# Autodesk Inventor part: 主动轮锥齿轮
Saved by Autodesk Inventor 2015 (Build 190159000, 159)
## iProperties
Created: 2017-06-08
Part Number: 主动轮锥齿轮
Material: 铝 6061
Document SubType Name: Modeling
Designer: Administrator
Categories: <?xml version="1.0" encoding="UTF-16"?> <MemberInstance><Categories><FamilyTemplate><FamilyTemplateParameter ValueType="xs:double" Id="1" ObjectReferenceKey="da_z" ObjectType="kUserParameterObject"/><FamilyTemplateParameter ValueType="xs:double" Id="2" ObjectReferenceKey="da_b" ObjectType="kUserParameterObject"/><FamilyTemplateParameter ValueType="xs:double" Id="3" ObjectReferenceKey="da_beta" ObjectType="kUserParameterObject"/><FamilyTemplateParameter ValueType="xs:double" Id="4" ObjectReferenceKey="da_dae" ObjectType="kUserParameterObject"/><FamilyTemplateParameter ValueType="xs:double" Id="5" ObjectReferenceKey="da_ve" ObjectType="kUserParameterObject"/><FamilyTemplateParameter ValueType="xs:double" Id="6" ObjectReferenceKey="da_omega" ObjectType="kUserParameterObject"/><FamilyTemplateParameter ValueType="xs:string" Id="7" ObjectReferenceKey="EAIAABAAAAAAHwAAAAAAAIAAAAAAAAAA" ObjectType="83914240" SubObjectId="SurfaceGeometry"/></FamilyTemplate><ParamToTemplateMap><ParamToTemplate CategoryParameter="//CategoryParameter[@InternalName='046C89C9-8512-4d59-83FE-43B91F4F132A']" TemplateParameter="1"/><ParamToTemplate CategoryParameter="//CategoryParameter[@InternalName='2552DF32-E462-4b46-AEBF-C6C7768E72AC']" TemplateParameter="2"/><ParamToTemplate CategoryParameter="//CategoryParameter[@InternalName='C9EE641D-15FC-4fae-A226-E94C4372FDD7']" TemplateParameter="3"/><ParamToTemplate><ParamToTemplate CategoryParameter="//CategoryParameter[@InternalName='00B6519A-459B-49c7-AD84-2E56D39A5744']" ConstantValue="0.000000"/></ParamToTemplate><ParamToTemplate><ParamToTemplate CategoryParameter="//CategoryParameter[@InternalName='04B31F0E-C7A6-4894-AA32-9629BEFACF47']" ConstantValue="1.000000"/></ParamToTemplate><ParamToTemplate><ParamToTemplate CategoryParameter="//CategoryParameter[@InternalName='43CBEC2E-7847-49e7-A936-2F7889FCB2D9']" ConstantValue="0.200000"/></ParamToTemplate><ParamToTemplate><ParamToTemplate CategoryParameter="//CategoryParameter[@InternalName='B1EFC894-105D-4ebd-86BF-FA20ED196853']" ConstantValue="0.300000"/></ParamToTemplate><ParamToTemplate><ParamToTemplate CategoryParameter="//CategoryParameter[@InternalName='51175063-3D10-4879-93E8-6246FE8B403D']" ConstantValue="2060000000.000000"/></ParamToTemplate><ParamToTemplate><ParamToTemplate CategoryParameter="//CategoryParameter[@InternalName='A3A52E27-4454-46a9-B0BD-C932399B70AF']" ConstantValue="0.300000"/></ParamToTemplate><ParamToTemplate CategoryParameter="//CategoryParameter[@InternalName='2A200944-5A8C-41ca-B96E-8520D2E510F1']" TemplateParameter="4"/><ParamToTemplate><ParamToTemplate CategoryParameter="//CategoryParameter[@InternalName='1A637F62-92C8-44bc-B81F-10802510B579']" ConstantValue="10.922917"/></ParamToTemplate><ParamToTemplate CategoryParameter="//CategoryParameter[@InternalName='B52DD4BE-6863-48fb-BF58-89EF6F9EC65C']" TemplateParameter="5"/><ParamToTemplate><ParamToTemplate CategoryParameter="//CategoryParameter[@InternalName='3956BFF2-84D2-457d-93C2-9B0613DEBA67']" ConstantValue="1.630592"/></ParamToTemplate><ParamToTemplate CategoryParameter="//CategoryParameter[@InternalName='739CFA02-461B-4bf8-8049-181FCAD8B28F']" TemplateParameter="6"/><ParamToTemplate><ParamToTemplate CategoryParameter="//CategoryParameter[@InternalName='A27E999F-E2CE-4481-8A2A-EBF499C4C3C5']" ConstantValue="0.000000"/></ParamToTemplate><ParamToTemplate><ParamToTemplate CategoryParameter="//CategoryParameter[@InternalName='9E1B4470-B2D3-4ff1-B813-535BB4CDF51A']" ConstantValue="3520000.000000"/></ParamToTemplate><ParamToTemplate><ParamToTemplate CategoryParameter="//CategoryParameter[@InternalName='F8452263-BFF6-458c-9FB1-07C4B99E95CD']" ConstantValue="11400000.000000"/></ParamToTemplate><ParamToTemplate><ParamToTemplate CategoryParameter="//CategoryParameter[@InternalName='3E3BB259-FD49-497f-8171-6EBC954A3479']" ConstantValue="2.000000"/></ParamToTemplate><ParamToTemplate CategoryParameter="//CategoryParameter[@InternalName='27C3BAF2-7550-4e4b-AE2C-0DB134B7D9B7']" TemplateParameter="7"/></ParamToTemplateMap><Category DisplayName="Gear" InternalName="DC85795E-93AB-48d5-8EEE-5A27447B64BD" Mnemonic="Gear"><CategoryParameter DisplayName="z" InternalName="046C89C9-8512-4d59-83FE-43B91F4F132A" Mnemonic="z"/><CategoryParameter DisplayName="b" InternalName="2552DF32-E462-4b46-AEBF-C6C7768E72AC" Mnemonic="b"/><CategoryParameter DisplayName="||b|" InternalName="C9EE641D-15FC-4fae-A226-E94C4372FDD7" Mnemonic="beta"/><CategoryParameter DisplayName="x" InternalName="00B6519A-459B-49c7-AD84-2E56D39A5744" Mnemonic="x"/><CategoryParameter DisplayName="a*" InternalName="04B31F0E-C7A6-4894-AA32-9629BEFACF47" Mnemonic="a"/><CategoryParameter DisplayName="c*" InternalName="43CBEC2E-7847-49e7-A936-2F7889FCB2D9" Mnemonic="c"/><CategoryParameter DisplayName="r|.f|*" InternalName="B1EFC894-105D-4ebd-86BF-FA20ED196853" Mnemonic="rf"/><CategoryParameter DisplayName="E" InternalName="51175063-3D10-4879-93E8-6246FE8B403D" Mnemonic="E"/><CategoryParameter DisplayName="||m|" InternalName="A3A52E27-4454-46a9-B0BD-C932399B70AF" Mnemonic="mi"/><Category DisplayName="BevelGear" InternalName="0C98F69A-0C2B-4791-B2FE-7691BB227E77" Mnemonic="BevelGear"><CategoryParameter DisplayName="d|.ae|" InternalName="2A200944-5A8C-41ca-B96E-8520D2E510F1" Mnemonic="dae"/><CategoryParameter DisplayName="d|.ai|" InternalName="1A637F62-92C8-44bc-B81F-10802510B579" Mnemonic="dai"/><CategoryParameter DisplayName="A|.e|" InternalName="B52DD4BE-6863-48fb-BF58-89EF6F9EC65C" Mnemonic="ve"/><CategoryParameter DisplayName="A|.i|" InternalName="3956BFF2-84D2-457d-93C2-9B0613DEBA67" Mnemonic="vi"/><CategoryParameter DisplayName="||S|" InternalName="739CFA02-461B-4bf8-8049-181FCAD8B28F" Mnemonic="omega"/><CategoryParameter DisplayName="x|.t|" InternalName="A27E999F-E2CE-4481-8A2A-EBF499C4C3C5" Mnemonic="xt"/><CategoryParameter DisplayName="||s||.Flim|" InternalName="9E1B4470-B2D3-4ff1-B813-535BB4CDF51A" Mnemonic="sFlim"/><CategoryParameter DisplayName="||s||.Hlim|" InternalName="F8452263-BFF6-458c-9FB1-07C4B99E95CD" Mnemonic="sHlim"/><CategoryParameter DisplayName="类型" InternalName="3E3BB259-FD49-497f-8171-6EBC954A3479" Mnemonic="type"/><CategoryParameter DisplayName="PitchDiameter" InternalName="27C3BAF2-7550-4e4b-AE2C-0DB134B7D9B7" Mnemonic="IDS_PITCHDIAM"/></Category></Category></Categories></MemberInstance>
Mass: 60.9118 g
Surface Area: 34.3074 cm^2
Volume: 7.7496 cm^3
Density: 2.7 g/cm^3
Appearance: 铝 - 平面
CustomPartVersion: 1
Author: Administrator
Autodesk Inventor part; units mm, degrees
ref_plane "网格平面 2" through (0, 0, 0) normal (0.9986295, 0.052336, 0) x (0, 0, 1)
sketch "齿实体草图" plane through (0, 0, 0) normal (1, 0, 0) x (0, 1, 0)
  line L0 (0, 0) -> (88.8616, -33.4153) construction
  line L1 (88.8616, -33.4153) -> (90.9487, -27.154)
  line L2 (90.9487, -27.154) -> (0, 0) construction
  line L3 (90, -30) -> (0, 0) construction
  line L4 (53.3613, -20.0658) -> (54.6146, -16.3059)
  line L5 (88.8616, -33.4153) -> (53.3613, -20.0658)
  line L6 (90.9487, -27.154) -> (54.6146, -16.3059)
  line L7 (0, -39.3868) -> (0, 6.5645) projected
  line L8 (0, -30) -> (90.9487, -30) construction
  dimension "d0" = 180
  dimension "d1" = 177.7232
  dimension "d2" = 181.8974
  dimension "d3" = 37.9
  dimension "d4" = 27.1539
  constraints: 16 end point, 4 point on line, 3 perpendicular, 2 collinear, 1 horizontal alignment, 1 vertical alignment
  measures "d0" diameter of L3.start L7
  measures "d1" diameter of L0.end L7
  measures "d2" diameter of L1.end L7
  measures "d3" distance between parallel lines of L1 L4
  measures "d4" vertical distance of L1.end L0.start
revolve "齿实体" add sketch "齿实体草图" angle 360 about axis through (0, 0, 0) along (0, 0, 1)
ref_plane "齿平面" through (0, 90, -30) normal (0, -0.9486833, 0.3162278) x (1, 0, 0)
sketch "起始草图" plane through (0, 90, -30) normal (0, -0.9486833, 0.3162278) x (1, 0, 0)
  line L0 (0, -23.5051) -> (0, 10.6448) projected
  arc A0 (-0.9303, -4.392) -> (-4.308, 4.948) centre (-95.025, -33.1399) ccw
  arc A1 (4.308, 4.948) -> (0.9303, -4.392) centre (95.025, -33.1399) ccw
  line L1 (-0.9303, -4.392) -> (0.9303, -4.392)
  arc A2 (4.308, 4.948) -> (-4.308, 4.948) centre (0, -284.605) ccw
  dimension "d7" = 98.3882
  dimension "d8" = 95.025
  dimension "d9" = 251.4651
  dimension "d57" = 289.585
  dimension "d58" = 280.213
  constraints: 6 point on circle, 3 centre point, 3 symmetric about line, 2 end point, 1 coincident, 1 perpendicular, 1 other
  measures "d7" radius of A0
  measures "d8" horizontal distance of point (0, -284.605) A0.centre
  measures "d9" vertical distance of point (0, -284.605) A0.centre
  measures "d57" radius of A2
  measures "d58" distance from line of A2.centre L1
ref_plane "终止平面" through (0, 53.7318, -17.9106) normal (0, -0.9486833, 0.3162278) x (1, 0, 0)
sketch "终止草图" plane through (0, 53.7318, -17.9106) normal (0, -0.9486833, 0.3162278) x (1, 0, 0)
  line L0 (0, -15.3589) -> (0, 6.9827) projected
  arc A0 (-0.5563, -2.3419) -> (-2.5763, 3.2436) centre (-56.8269, -19.5337) ccw
  arc A1 (2.5763, 3.2436) -> (0.5563, -2.3419) centre (56.8269, -19.5337) ccw
  line L1 (-0.5563, -2.3419) -> (0.5563, -2.3419)
  arc A2 (2.5763, 3.2436) -> (-2.5763, 3.2436) centre (0, -169.915) ccw
  dimension "d12" = 58.8382
  dimension "d15" = 56.8269
  dimension "d16" = 150.3813
  dimension "d59" = 173.1777
  dimension "d60" = 167.5731
  constraints: 6 point on circle, 3 centre point, 3 symmetric about line, 2 end point, 1 coincident, 1 other
  measures "d12" radius of A0
  measures "d15" horizontal distance of A0.centre point (0, -169.915)
  measures "d16" vertical distance of A0.centre point (0, -169.915)
  measures "d59" radius of A2
  measures "d60" distance from line of A2.centre L1
loft "Loft" cut profiles "起始草图", "终止草图"
pattern_circular "Circular Pattern" count 60 over 360 about axis through (0, 0, 0) along (0, 0, 1) of "Loft"
sketch3d "三维草图 (右)"
ref_plane "终止平面 (右)" through (-10.3164, 52.7322, -17.9106) normal (0.1821455, -0.9310333, 0.3162278) x (0.9813953, 0.1919982, 0)
sketch "终止草图 (右)" plane through (-10.3164, 52.7322, -17.9106) normal (0.1821455, -0.9310333, 0.3162278) x (0.9813953, 0.1919982, 0)
  arc A0 (-0.5563, -2.3419) -> (-2.5763, 3.2436) centre (-56.8269, -19.5337) ccw
  line L0 (0, -205.7571) -> (0, 39.6332) projected
  arc A1 (2.5763, 3.2436) -> (0.5563, -2.3419) centre (56.8269, -19.5337) ccw
  line L1 (-0.5563, -2.3419) -> (0.5563, -2.3419)
  arc A2 (2.5763, 3.2436) -> (-2.5763, 3.2436) centre (0, -169.915) ccw
  dimension "d70" = 56.8269
  dimension "d71" = 150.3813
  dimension "d72" = 58.8382
  dimension "d73" = 167.5731
  dimension "d74" = 173.1777
  constraints: 6 point on circle, 3 centre point, 3 symmetric about line, 2 end point, 1 coincident, 1 perpendicular, 1 other
  measures "d70" horizontal distance of A2.centre A0.centre
  measures "d71" vertical distance of point (0, -169.915) A0.centre
  measures "d72" radius of A0
  measures "d73" distance from line of point (0, -169.915) L1
  measures "d74" radius of A2
feature "放样 (右)" [suppressed]
pattern_circular "环形阵列 (右)" [suppressed]
sketch3d "三维草图 (左)"
ref_plane "终止平面 (左)" through (10.4643, 52.7322, -18.0384) normal (-0.1845365, -0.9299226, 0.3181041) x (0.9808733, -0.1946473, 0)
sketch "终止草图 (左)" plane through (10.4643, 52.7322, -18.0384) normal (-0.1845365, -0.9299226, 0.3181041) x (0.9808733, -0.1946473, 0)
  line L0 (0, -206.7579) -> (0, 40.7486) projected
  arc A0 (-0.5563, -2.2295) -> (-2.5763, 3.356) centre (-56.8269, -19.4213) ccw
  arc A1 (2.5763, 3.356) -> (0.5563, -2.2295) centre (56.8269, -19.4213) ccw
  line L1 (-0.5563, -2.2295) -> (0.5563, -2.2295)
  ellipse E0 centre (0, -15.4589) end of major axis (54.6146, -15.4589) minor radius 17.3731 projected
  arc A2 (2.5763, 3.356) -> (-2.5763, 3.356) centre (0, -169.8026) ccw
  dimension "d56" = 17.3731
  dimension "d30" = 58.8382
  dimension "d31" = 56.8269
  dimension "d32" = 150.3813
  dimension "d61" = 173.1777
  dimension "d62" = 167.5731
  constraints: 6 point on circle, 3 centre point, 3 symmetric about line, 2 end point, 1 coincident, 2 other
  measures "d30" radius of A0
  measures "d31" horizontal distance of point (0, -169.803) A0.centre
  measures "d32" vertical distance of A0.centre point (0, -169.803)
  measures "d61" radius of A2
  measures "d62" distance from line of point (0, -169.803) L1
feature "放样 (左)" [suppressed]
pattern_circular "环形阵列 (左)" [suppressed]
sketch "实体草图" plane through (0, 0, 0) normal (1, 0, 0) x (0, 1, 0)
  line L0 (0, -35.0375) -> (0, -19.5308) projected
  line L1 (88.8616, -33.4153) -> (53.3613, -20.0658) projected
  line L2 (53.3613, -20.0658) -> (0, -20.0658)
  line L3 (88.8616, -33.4153) -> (0, -33.4153)
  constraints: 4 end point, 2 perpendicular, 2 point on line
revolve "固定实体" add sketch "实体草图" angle 360 about axis through (0, 0, 0) along (0, 0, 1)
sketch "Sketch6" plane through (0, 0, 0) normal (1, 0, 0) x (0, 1, 0)
  line L0 (90, -30) -> (0, 0) projected
  line L1 (0, -37.7999) -> (0, 6.3) projected
surface revolve "中径" sketch "Sketch6" angle 360 about axis through (0, 0, 0) along (0, 0, 1) shown no curves L0
equation "\"d0\" = da_de"
equation "\"d1\" = da_dfe"
equation "\"d2\" = da_dae"
equation "\"d3\" = da_b"
equation "\"d4\" = da_ve"
equation "\"d7\" = fd_rr"
equation "\"d8\" = fd_x"
equation "\"d9\" = fd_y"
equation "\"d57\" = 0.5 * fd_dva + 0.3 * da_he"
equation "\"d58\" = 0.5 * fd_dva - 1.12 * da_he"
equation "\"da_teethtype\" = 0"
equation "\"da_b\" = 37.9"
equation "\"da_de\" = 180"
equation "\"da_dae\" = 181.89737"
equation "\"da_dfe\" = 177.72316"
equation "\"da_le\" = 94.86833"
equation "\"da_omega\" = 90deg"
equation "\"da_beta\" = 0"
equation "\"da_delta\" = 71.565051deg"
equation "\"da_alpha\" = 20deg"
equation "\"da_he\" = 6.6"
equation "\"da_ve\" = 27.15395"
equation "\"da_zv\" = 189.73666"
equation "\"fd_loft\" = da_b + 0.05 * da_he"
equation "\"fd_x\" = fd_x1 + fd_x2"
equation "\"fd_y\" = fd_y1 - fd_y2"
equation "\"fd_dd\" = fd_dva - 0.8 * da_he"
equation "\"da_dvw\" = 569.20998"
equation "\"d11\" = fd_loft"
equation "\"da_dm\" = 144.0449"
equation "\"da_x\" = 0"
equation "\"da_m\" = 3"
equation "\"d50\" = da_omega"
equation "\"fd_rr\" = 98.388237"
equation "\"fd_dva\" = 575.209979"
equation "\"fd_x1\" = 2.382347"
equation "\"fd_x2\" = 92.64262"
equation "\"fd_y1\" = 284.595018"
equation "\"fd_y2\" = 33.129899"
body "Solid1"
body "Srf1"
